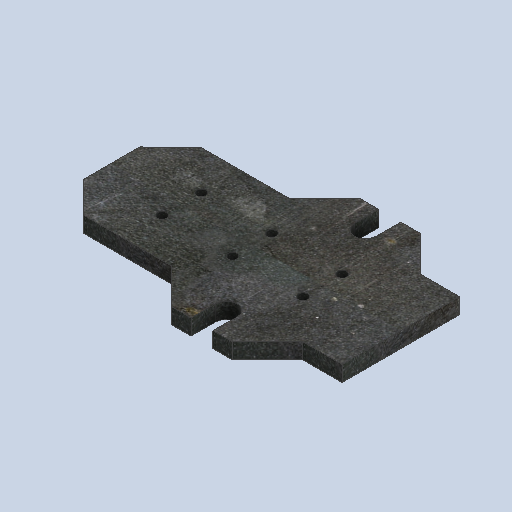
# Autodesk Inventor part: Grundplatte
Saved by Autodesk Inventor 2023.2 (Build 272271000, 271)
## iProperties
Created: 2023-02-07
Part Number: Grundplatte
Material: Steel
Document SubType Name: Modeling
Designer: Ayush
Density: 7.85 g/cm^3
Appearance: Plate
Author: Ayush
Autodesk Inventor part; units mm, degrees
ref_plane "YZ Plane" through (0, 0, 0) normal (1, 0, 0) x (0, 1, 0)
ref_plane "XZ Plane" through (0, 0, 0) normal (0, 1, 0) x (-1, 0, 0)
ref_plane "XY Plane" through (0, 0, 0) normal (0, 0, 1) x (1, 0, 0)
sketch "Sketch1" plane through (0, 0, 0) normal (0, 1, 0) x (-1, 0, 0)
  line L0 (184.4366, -17.5) -> (184.4366, 17.5)
  line L1 (184.4366, -17.5) -> (164.4366, -37.5)
  line L2 (184.4366, -17.5) -> (247.2296, -17.5) construction
  line L3 (184.4366, 17.5) -> (164.4366, 37.5)
  line L4 (184.4366, 17.5) -> (233.0996, 17.5) construction
  line L5 (-0.5634, 37.5) -> (-0.5634, -37.5)
  arc A0 (59.4366, 44.5) -> (73.4366, 44.5) centre (66.4366, 44.5) ccw
  arc A1 (73.4366, -44.5) -> (59.4366, -44.5) centre (66.4366, -44.5) ccw
  line L6 (39.6866, 60) -> (27.1866, 60)
  line L7 (59.4366, 44.5) -> (59.4366, 60)
  line L8 (73.4366, 44.5) -> (73.4366, 60)
  line L9 (73.4366, -44.5) -> (73.4366, -60)
  line L10 (59.4366, -44.5) -> (59.4366, -60)
  line L11 (59.4366, 60) -> (46.9366, 60)
  line L12 (46.9366, 60) -> (24.4366, 37.5)
  line L13 (59.4366, -60) -> (46.9366, -60)
  line L14 (46.9366, -60) -> (24.4366, -37.5)
  line L15 (73.4366, 60) -> (85.9366, 60)
  line L16 (85.9366, 60) -> (108.4366, 37.5)
  line L17 (85.9366, 60) -> (117.7565, 60) construction
  line L18 (73.4366, -60) -> (85.9366, -60)
  line L19 (85.9366, -60) -> (108.4366, -37.5)
  line L20 (164.4366, -37.5) -> (108.4366, -37.5)
  line L21 (24.4366, -37.5) -> (-0.5634, -37.5)
  line L22 (164.4366, 37.5) -> (108.4366, 37.5)
  line L23 (24.4366, 37.5) -> (-0.5634, 37.5)
  circle A2 centre (139.4366, 12.5) radius 5.5
  circle A3 centre (139.4366, -12.5) radius 5.5
  circle A4 centre (94.4366, -12.5) radius 5.5
  circle A5 centre (94.4366, 12.5) radius 5.5
  circle A6 centre (49.4366, 12.5) radius 5.5
  circle A7 centre (49.4366, -12.5) radius 5.5
  point P0 (0, 0)
  point P1 (-0.5634, 0)
  dimension "d4" = 35
  dimension "d5" = 135
  dimension "d7" = 135
  dimension "d9" = 185
  dimension "d10" = 75
  dimension "d19" = 14
  dimension "d20" = 14
  dimension "d23" = 67
  dimension "d24" = 67
  dimension "d27" = 12.5
  dimension "d28" = 15.5
  dimension "d29" = 15.5
  dimension "d30" = 15.5
  dimension "d31" = 15.5
  dimension "d32" = 12.5
  dimension "d33" = 135
  dimension "d34" = 12.5
  dimension "d35" = 135
  dimension "d36" = 12.5
  dimension "d37" = 45
  dimension "d38" = 12.5
  dimension "d39" = 135
  dimension "d40" = 11
  dimension "d41" = 11
  dimension "d42" = 11
  dimension "d43" = 11
  dimension "d44" = 11
  dimension "d45" = 11
  dimension "d46" = 50
  dimension "d47" = 45
  dimension "d48" = 45
  dimension "d49" = 25
  constraints: 48 end point, 12 horizontal, 8 centre point, 4 horizontal alignment, 4 point on circle, 4 tangent, 4 vertical, 3 vertical alignment, 2 perpendicular, 1 equal length, 1 midpoint, 1 parallel
  measures "d4" distance of L0.start L0.end
  measures "d5" angle of L1 L2
  measures "d7" angle of L4 L3
  measures "d9" distance between parallel lines of L5 L0
  measures "d10" distance of L5.end L5.start
  measures "d19" diameter of A0
  measures "d20" diameter of A1
  measures "d23" distance from line of L5 A0.centre
  measures "d24" distance from line of L5 A1.centre
  measures "d27" distance of L6.start L6.end
  measures "d28" distance of L7.start L7.end
  measures "d29" distance of L8.start L8.end
  measures "d30" distance of L9.start L9.end
  measures "d31" distance of L10.start L10.end
  measures "d32" distance of L7.end L11.end
  measures "d33" angle of L12 L11
  measures "d34" distance of L10.end L13.end
  measures "d35" angle of L13 L14
  measures "d36" distance of L8.end L15.end
  measures "d37" angle of L16 L17
  measures "d38" distance of L9.end L18.end
  measures "d39" angle of L19 L18
  measures "d40" diameter of A2
  measures "d41" diameter of A3
  measures "d42" diameter of A4
  measures "d43" diameter of A5
  measures "d44" diameter of A6
  measures "d45" diameter of A7
  measures "d46" distance from line of A7.centre L5
  measures "d47" distance of A4.centre A7.centre
  measures "d48" distance of A3.centre A4.centre
  measures "d49" distance of A7.centre A6.centre
extrude "Extrusion1" add sketch "Sketch1" along normal blind 6
sketch "Sketch2" plane through (0, 6, 0) normal (0, 1, 0) x (1, 0, 0)
  line L0 (-108.4366, 37.5) -> (-164.4366, 37.5) projected
  line L1 (-164.4366, 37.5) -> (-108.4366, 37.5)
  line L2 (-73.4366, 60) -> (-85.9366, 60) projected
  line L3 (-108.4366, 37.5) -> (-85.9366, 60)
  line L4 (-85.9366, 60) -> (-73.4366, 60)
  arc A0 (-73.4366, 44.5) -> (-59.4366, 44.5) centre (-66.4366, 44.5) ccw projected
  line L5 (-73.4366, 60) -> (-73.4366, 44.5)
  line L6 (-164.4366, 37.5) -> (-184.4366, 18.1375)
  line L7 (-184.4366, 17.5) -> (-184.4366, -17.5) projected
  line L8 (-184.4366, 18.1375) -> (-184.4366, -17.5)
  line L9 (-184.4366, -17.5) -> (-164.4366, -37.5)
  line L10 (-184.4366, -17.5) -> (-164.4366, -37.5) projected
  line L11 (-164.4366, -37.5) -> (-108.4366, -37.5) projected
  line L12 (-108.802, -37.5) -> (-85.9366, -60)
  line L13 (-108.4366, -37.5) -> (-85.9366, -60) projected
  line L14 (-85.9366, -60) -> (-73.4366, -60) projected
  line L15 (-73.4366, -60) -> (-73.4366, -44.5) projected
  line L16 (-73.4366, -60) -> (-73.4366, -44.5)
  line L17 (-59.4366, -44.5) -> (-59.4366, -60) projected
  line L18 (-59.4366, -44.5) -> (-59.4366, -60)
  line L19 (-59.4366, -60) -> (-46.9366, -60) projected
  line L20 (-59.4366, -60) -> (-46.9366, -60)
  line L21 (-46.9366, -60) -> (-24.4366, -37.5)
  line L22 (-46.9366, -60) -> (-24.4366, -37.5) projected
  line L23 (-24.4366, -37.5) -> (0.5634, -37.5) projected
  line L24 (0.5634, -37.5) -> (0.5634, 37.5) projected
  line L25 (0.5634, -37.5) -> (0.5634, 37.5)
  line L26 (0.5634, 37.5) -> (-24.4366, 37.5) projected
  line L27 (0.5634, 37.5) -> (-24.4366, 37.5)
  line L28 (-24.4366, 37.5) -> (-46.9366, 60)
  line L29 (-59.4366, 60) -> (-59.4366, 44.5) projected
  line L30 (-46.9366, 60) -> (-59.4366, 60)
  line L31 (-59.4366, 60) -> (-59.4366, 44.5)
  arc A1 (-59.4366, -44.5) -> (-73.4366, -44.5) centre (-66.4366, -44.5) ccw
  arc A2 (-73.4366, 44.5) -> (-59.4366, 44.5) centre (-66.4366, 44.5) ccw
  circle A3 centre (-139.4366, 12.5) radius 3
  circle A4 centre (-139.4366, -12.5) radius 3
  circle A5 centre (-94.4366, -12.5) radius 3
  circle A6 centre (-94.4366, 12.5) radius 3
  circle A7 centre (-49.4366, 12.5) radius 3
  circle A8 centre (-49.4366, -12.5) radius 3
  point P0 (0, 0)
  dimension "d53" = 14
  dimension "d55" = 6
  dimension "d56" = 6
  dimension "d57" = 6
  dimension "d58" = 6
  dimension "d59" = 6
  dimension "d60" = 6
  dimension "d61" = 50
  dimension "d62" = 45
  dimension "d63" = 45
  dimension "d64" = 12.5
  dimension "d65" = 25
  constraints: 37 end point, 8 centre point, 8 collinear, 5 coincident, 4 horizontal alignment, 4 point on circle, 3 perpendicular, 1 parallel, 1 point on line, 1 tangent, 1 vertical alignment
  measures "d53" diameter of A1
  measures "d55" diameter of A3
  measures "d56" diameter of A4
  measures "d57" diameter of A5
  measures "d58" diameter of A6
  measures "d59" diameter of A7
  measures "d60" diameter of A8
  measures "d61" distance from line of A7.centre L24
  measures "d62" distance of A6.centre A7.centre
  measures "d63" distance of A3.centre A6.centre
  measures "d64" vertical distance of A7.centre point (0, 0)
  measures "d65" distance of point (-49.437, -12.5) A7.centre
extrude "Extrusion2" add sketch "Sketch2" along normal blind 4 contours L3 L2 L5 A0 L29 L30 L28 L26 L24 L23 L21 L19 L17 A1 L15 L14 L13 L11 L9 L7 L8 L6 L0
body "Solid1"
